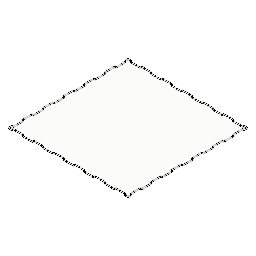
TopPlate v10 (Autodesk Fusion 360 design; units mm, degrees)
Autodesk Fusion 360 part; units mm, degrees
sketch "Sketch1" plane through (0, 0, 0) normal (0, 0, 1) x (1, 0, 0)
  line L0 (0, 0) -> (350, 0)
  line L1 (350, 0) -> (350, 350)
  line L2 (350, 350) -> (0, 350)
  line L3 (0, 350) -> (0, 0)
  point P0 (175, 175)
  dimension "d1" = 350
  dimension "d2" = 350
  dimension "d7" = 175
  dimension "d8" = 175
  constraint horizontal L0
  constraint vertical L1
  constraint horizontal L2
  constraint vertical L3
  constraint coincident L0.start L3.end
  measures "d1" distance of L0.start L0.end
  measures "d2" distance of L0.start L2.end
  measures "d7" distance of L0 P0
  measures "d8" distance of L1 P0
extrude "Extrude1" add sketch "Sketch1" along normal blind 4 makes body 1
sketch "Sketch2" plane through (0, 0, 4) normal (0, 0, 1) x (-1, 0, 0)
  line L0 (0, -350) -> (0, 0)
  line L1 (-10, 0) -> (-40, 0)
  line L2 (-40, 0) -> (-40, -4)
  line L3 (-40, -4) -> (-10, -4)
  line L4 (-10, -4) -> (-10, 0)
  line L5 (0, -10) -> (-4, -10)
  line L6 (-4, -10) -> (-4, -40)
  line L7 (-4, -40) -> (0, -40)
  line L8 (0, -40) -> (0, -10)
  line L9 (0, 0) -> (-350, 0)
  dimension "d12" = 10
  dimension "d14" = 30
  dimension "d15" = 4
  dimension "d26" = 30
  dimension "d27" = 4
  dimension "d47" = 10
  constraint horizontal L1
  constraint vertical L2
  constraint horizontal L3
  constraint vertical L4
  constraint horizontal L5
  constraint vertical L6
  constraint horizontal L7
  constraint vertical L8
  constraint coincident L0 L5.start
  constraint coincident L1.end L9
  measures "d12" distance of L0 L4
  measures "d14" distance of L2.end L3.end
  measures "d15" distance of L1.end L2.end
  measures "d26" distance of L5.end L6.end
  measures "d27" distance of L6.end L7.end
  measures "d47" distance of L5 L9
extrude "Extrude4" cut sketch "Sketch2" against normal through all contours L0 L5 L6 L7 L8 bodies 1
extrude "Extrude5" cut sketch "Sketch2" against normal through all contours L1 L2 L3 L4 L9 bodies 1
pattern_linear "R-Pattern1" count 6 spacing 60 along (0, 1, 0) count 2 spacing 346 along (1, 0, 0) of "Extrude4"
pattern_linear "R-Pattern2" count 6 spacing 60 along (1, 0, 0) count 2 spacing 346 along (0, 1, 0) of "Extrude5"
copy_body "Body->Comp1" bodies 1 removing the originals makes body 2 in component "Component"
component "Component" placed x (1, 0, 0) y (0, 1, 0) z (0, 0, 1) at (0, 0, 0)
equation "d1 = Linear Dimension-2"
equation "mm = 툁"
equation "d2 = d"
equation "b = 350 mm" comment "width"
equation "d = 350 mm" comment "depth"
equation "h = 290 mm" comment "height"
equation "t = 4 mm" comment "thickness"
equation "d7 = d / 2"
equation "d8 = b / 2"
equation "d9 = t"
equation "a = 30 mm"
equation "d12 = b_corner"
equation "b_corner = ( b - ( floor(b / a) * a ) ) / 2"
equation "d14 = a"
equation "d15 = t"
equation "n_b = floor(floor(b / a) / 2) + 1"
equation "d26 = a"
equation "d27 = t"
equation "d_corner = ( d - ( floor(d / a) * a ) ) / 2"
equation "n_d = floor(floor(d / a) / 2) + 1"
equation "d39 = n_d"
equation "d41 = 2 * a"
equation "d42 = b - t"
equation "d43 = n_b"
equation "d45 = 2 * a"
equation "d46 = d - t"
equation "d47 = d_corner"
